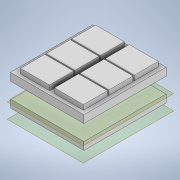
# Autodesk Inventor part: UberV2
Saved by Autodesk Inventor 2020 (Build 240168000, 168)
## iProperties
Created: 2020-02-16
Part Number: UberV2
Material: Generic
Document SubType Name: Modeling
Designer: atmat
Density: 1 g/cm^3
Appearance: Default
Author: atmat
Autodesk Inventor part; units mm, degrees
ref_plane "YZ Plane" through (0, 0, 0) normal (1, 0, 0) x (0, 1, 0)
ref_plane "XZ Plane" through (0, 0, 0) normal (0, 1, 0) x (-1, 0, 0)
ref_plane "XY Plane" through (0, 0, 0) normal (0, 0, 1) x (1, 0, 0)
sketch "Sketch1" plane through (0, 0, 0) normal (0, 1, 0) x (-1, 0, 0)
  line L0 (7.15, 8.5) -> (-7.15, 8.5)
  line L1 (-7.15, 8.5) -> (-7.15, -8.5)
  line L2 (-7.15, -8.5) -> (7.15, -8.5)
  line L3 (7.15, -8.5) -> (7.15, 8.5)
  point P0 (0, 0)
  dimension "d0" = 17
  dimension "d1" = 14.3
  dimension "d2" = 8.5
  dimension "d3" = 7.15
  constraints: 8 end point, 2 parallel, 1 horizontal, 1 perpendicular
  measures "d0" distance of L2.end L0.start
  measures "d1" distance of L1.end L2.end
  measures "d2" distance from line of point (0, 0) L2
  measures "d3" distance from line of point (0, 0) L3
extrude "Extrusion1" add sketch "Sketch1" along normal blind 1.6
sketch "Sketch2" plane through (0, 1.6, 0) normal (0, 1, 0) x (1, 0, 0)
  line L0 (-6.7, -7.75) -> (-0.7, -7.75)
  line L1 (-0.7, -7.75) -> (-0.7, -2.75)
  line L2 (-0.7, -2.75) -> (-6.7, -2.75)
  line L3 (-6.7, -2.75) -> (-6.7, -7.75)
  line L4 (-6.7, -2.5) -> (-0.7, -2.5)
  line L5 (-0.7, -2.5) -> (-0.7, 2.5)
  line L6 (-0.7, 2.5) -> (-6.7, 2.5)
  line L7 (-6.7, 2.5) -> (-6.7, -2.5)
  line L8 (-6.7, 2.75) -> (-0.7, 2.75)
  line L9 (-0.7, 2.75) -> (-0.7, 7.75)
  line L10 (-0.7, 7.75) -> (-6.7, 7.75)
  line L11 (-6.7, 7.75) -> (-6.7, 2.75)
  line L12 (-7.15, -8.5) -> (7.15, -8.5) projected
  line L13 (0.3, -7.75) -> (6.3, -7.75)
  line L14 (6.3, -7.75) -> (6.3, -2.75)
  line L15 (6.3, -2.75) -> (0.3, -2.75)
  line L16 (0.3, -2.75) -> (0.3, -7.75)
  line L17 (0.3, -2.5) -> (6.3, -2.5)
  line L18 (6.3, -2.5) -> (6.3, 2.5)
  line L19 (6.3, 2.5) -> (0.3, 2.5)
  line L20 (0.3, 2.5) -> (0.3, -2.5)
  line L21 (0.3, 2.75) -> (6.3, 2.75)
  line L22 (6.3, 2.75) -> (6.3, 7.75)
  line L23 (6.3, 7.75) -> (0.3, 7.75)
  line L24 (0.3, 7.75) -> (0.3, 2.75)
  line L25 (-7.15, 8.5) -> (-7.15, -8.5) projected
  point P0 (0, 0)
  dimension "d6" = 5
  dimension "d7" = 6
  dimension "d8" = 5
  dimension "d9" = 5
  dimension "d10" = 0.25
  dimension "d11" = 0.25
  dimension "d12" = 0.75
  dimension "d13" = 5
  dimension "d14" = 5
  dimension "d15" = 5
  dimension "d16" = 6
  dimension "d17" = 6
  dimension "d18" = 6
  dimension "d19" = 0.25
  dimension "d20" = 0.25
  dimension "d21" = 1
  dimension "d22" = 0.45
  constraints: 48 end point, 12 parallel, 6 horizontal, 6 perpendicular, 5 collinear, 2 point on line
  measures "d6" distance of L2.end L0.start
  measures "d7" distance of L1.end L2.end
  measures "d8" distance of L4.end L5.end
  measures "d9" distance of L10.end L8.start
  measures "d10" distance between parallel lines of L6 L8
  measures "d11" distance between parallel lines of L2 L4
  measures "d12" distance between parallel lines of L12 L0
  measures "d13" distance of L15.end L13.start
  measures "d14" distance of L19.end L17.start
  measures "d15" distance of L23.end L21.start
  measures "d16" distance of L13.start L13.end
  measures "d17" distance of L17.start L17.end
  measures "d18" distance of L21.start L21.end
  measures "d19" distance between parallel lines of L19 L21
  measures "d20" distance between parallel lines of L15 L17
  measures "d21" distance between parallel lines of L16 L1
  measures "d22" distance between parallel lines of L25 L3
extrude "Extrusion2" add sketch "Sketch2" along normal blind 1
ref_plane "Work Plane1" through (0, -3.2, 0) normal (0, -1, 0) x (1, 0, 0)
sketch "Sketch3" plane through (0, -3.2, 0) normal (0, -1, 0) x (1, 0, 0)
  line L0 (7.15, 8.5) -> (7.15, -8.5) projected
  line L1 (-7.15, -8.5) -> (-7.15, 8.5) projected
  line L2 (7.15, -8.5) -> (-7.15, -8.5)
  line L3 (-7.15, -8.5) -> (-7.15, 8.5)
  line L4 (-7.15, 8.5) -> (7.15, 8.5)
  line L5 (7.15, 8.5) -> (7.15, -8.5)
  point P0 (0, 0)
  constraints: 8 end point, 2 parallel, 1 horizontal, 1 perpendicular
extrude "Extrusion3" add sketch "Sketch3" along normal blind 1.6
ref_plane "Work Plane2" through (0, -6.3, 0) normal (0, -1, 0) x (1, 0, 0)
sketch "Sketch4" plane through (-7.15, 0, -8.5) normal (-1, 0, 0) x (0, 0, 1)
  line L0 (0, 0) -> (0, 1.6) projected
  line L1 (17, 0) -> (17, 1.6) projected
  line L2 (0, 0) -> (17, 0)
  line L3 (17, 0) -> (17, 1.6)
  line L4 (17, 1.6) -> (0, 1.6)
  line L5 (0, 1.6) -> (0, 0)
  point P0 (8.5, 0)
  constraints: 8 end point, 2 parallel, 1 horizontal, 1 perpendicular
extrude "Extrusion4" add sketch "Sketch4" along normal blind 0.89
sketch "Sketch5" plane through (-7.15, -3.2, -8.5) normal (-1, 0, 0) x (0, 0, 1)
  line L0 (0, 0) -> (0, -1.6) projected
  line L1 (0, -1.6) -> (17, -1.6)
  line L2 (17, -1.6) -> (17, 0)
  line L3 (17, 0) -> (0, 0)
  line L4 (0, 0) -> (0, -1.6)
  point P0 (8.5, 3.2)
  constraints: 8 end point, 2 parallel, 1 horizontal, 1 perpendicular
extrude "Extrusion5" add sketch "Sketch5" along normal blind 0.89
body "Solid1"
